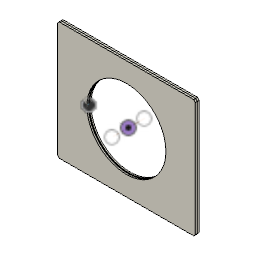
assembly (Autodesk Fusion 360 archive; units mm, degrees)
design "Condensor lens mount"
part number: 2026-06-29-18-31-42-518
Autodesk Fusion 360 part; units mm, degrees
sketch "Sketch1" plane through (0, 0, 0) normal (0, 1, 0) x (1, 0, 0)
  line L0 (87.5, -75) -> (-87.5, -75)
  line L1 (-87.5, -75) -> (-87.5, 75)
  line L2 (-87.5, 75) -> (87.5, 75)
  line L3 (87.5, 75) -> (87.5, -75)
  line L4 (87.5, -75) -> (-87.5, 75) construction
  line L5 (-87.5, -75) -> (87.5, 75) construction
  line L6 (-87.5, -72.7222) -> (-85.5476, -75)
  line L7 (0, -75) -> (0, 75) construction
  line L8 (-87.5, 0) -> (87.5, 0) construction
  line L9 (87.5, -72.7222) -> (85.5476, -75)
  line L10 (87.5, 72.7222) -> (85.5476, 75)
  line L11 (-87.5, 72.7222) -> (-85.5476, 75)
  circle A0 centre (0, 0) radius 50
  dimension "d1" = 175
  dimension "d2" = 150
  dimension "d3" = 3
  dimension "d4" = 100
  constraint horizontal L0
  constraint perpendicular L0 L1
  constraint parallel L0 L2
  constraint parallel L1 L3
  constraint coincident L4 A0.centre
  constraint coincident L5 A0.centre
  constraint coincident A0.centre origin
  constraint coincident L1 L6.start
  constraint coincident L0 L6.end
  constraint perpendicular L5 L6
  constraint midpoint L0 L7.start
  constraint midpoint L2 L7.end
  constraint midpoint L1 L8.start
  constraint midpoint L3 L8.end
  constraint symmetric L6.start L7 L9.start
  constraint symmetric L6.end L7 L9.end
  constraint symmetric L6.start L8 L11.start
  constraint symmetric L6.end L8 L11.end
  constraint symmetric L8 L9.start L10.start
  constraint symmetric L8 L9.end L10.end
  measures "d1" distance of L1.end L2.end
  measures "d2" distance of L0.end L1.end
  measures "d3" distance of L6.start L6.end
  measures "d4" diameter of A0
sketch "Sketch2" plane through (0, 2.5, 0) normal (0, 1, 0) x (1, 0, 0)
sketch "Sketch3" plane through (50, 2.5597, 0) normal (-1, 0, 0) x (0, -1, 0)
sketch "Sketch5" plane through (0, 0, 0) normal (0, 0, 1) x (1, 0, 0)
  line L0 (-50, 0.5) -> (-50, -0.5)
  arc A0 (-50, 0.5) -> (-50, -0.5) centre (-50, 0) ccw
  line L1 (0, 20) -> (0, -21)
  line L2 (-50.5, 0) -> (0, 0) construction
  dimension "d9" = 1
  dimension "d14" = 1
  constraint vertical L0
  constraint midpoint L0 A0.centre
  constraint vertical L1
  constraint midpoint A0 L2.start
  constraint coincident L2.end origin
  constraint perpendicular L1 L2
  measures "d9" distance of L0.start L0.end
  measures "d14" diameter of A0
extrude "Extrude4" add sketch "Sketch1" along normal mid plane 5 contours L0 L1 L2 L3 L6 L9 L10 L11 makes body 1
revolve "Revolve2" cut sketch "Sketch5" angle 360 about axis through (0, 20, 0) along (0, -1, 0) bodies 1
fillet "Fillet1" radius 0.1 2 edges at (-46.6164, 0.5, -18.0808) (-46.6164, -0.5, 18.0808) on bodies 1
split "Split1" by plane through (0, 0, 0) normal (0, 1, 0) bodies 1 makes body 2 at (75, 2.5, 0)

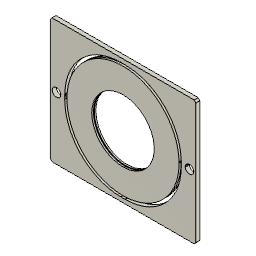
design "Projector Lens mount"
part number: 2026-06-30-17-54-35-923
part number: 2026-08-02-16-02-17-877
part number: 2026-08-02-16-06-35-428
Autodesk Fusion 360 part; units mm, degrees
sketch "Sketch1" plane through (0, 0, 0) normal (0, 1, 0) x (1, 0, 0)
  line L0 (87.5, -75) -> (-87.5, -75)
  line L1 (-87.5, -75) -> (-87.5, 75)
  line L2 (-87.5, 75) -> (87.5, 75)
  line L3 (87.5, 75) -> (87.5, -75)
  line L4 (87.5, -75) -> (-87.5, 75) construction
  line L5 (-87.5, -75) -> (87.5, 75) construction
  circle A0 centre (0, 0) radius 37.5
  line L6 (-87.5, -72.7222) -> (-85.5476, -75)
  line L7 (0, -75) -> (0, 75) construction
  line L8 (-87.5, 0) -> (87.5, 0) construction
  line L9 (87.5, -72.7222) -> (85.5476, -75)
  line L10 (-87.5, 72.7222) -> (-85.5476, 75)
  line L11 (87.5, 72.7222) -> (85.5476, 75)
  circle A1 centre (0, 0) radius 67.5
  line L12 (-69.3129, -70) -> (-70.6939, 70)
  line L13 (-81.6667, -70) -> (-82.5, -70)
  line L14 (-82.5, 70) -> (-81.6667, 70)
  line L15 (69.3129, -70) -> (70.6939, 70)
  line L16 (82.5, -70) -> (81.6667, -70)
  line L17 (69.3129, -70) -> (-69.3129, -70)
  line L18 (-70.6939, 70) -> (70.6939, 70)
  line L19 (81.6667, 70) -> (82.5, 70)
  dimension "d1" = 175
  dimension "d2" = 150
  dimension "d3" = 75
  dimension "d4" = 3
  dimension "d14" = 135
  dimension "d21" = 70
  constraint horizontal L0
  constraint perpendicular L0 L1
  constraint parallel L0 L2
  constraint parallel L1 L3
  constraint coincident L4 A0.centre
  constraint coincident L5 A0.centre
  constraint coincident A0.centre A1.centre
  constraint coincident L1 L6.start
  constraint coincident L0 L6.end
  constraint perpendicular L5 L6
  constraint midpoint L0 L7.start
  constraint midpoint L2 L7.end
  constraint midpoint L1 L8.start
  constraint midpoint L3 L8.end
  constraint symmetric L6.start L7 L9.start
  constraint symmetric L6.end L7 L9.end
  constraint symmetric L6.start L8 L10.start
  constraint symmetric L6.end L8 L10.end
  constraint symmetric L8 L9.start L11.start
  constraint symmetric L8 L9.end L11.end
  constraint concentric A0 A1
  constraint coincident L5 L13.start
  constraint collinear L13 L17
  constraint coincident L4 L14.end
  constraint collinear L14 L18
  constraint symmetric L7 L12.start L15.start
  constraint symmetric L7 L12.end L15.end
  constraint coincident L4 L16.end
  constraint collinear L16 L17
  constraint coincident L5 L19.start
  constraint collinear L18 L19
  measures "d1" distance of L1.end L2.end
  measures "d2" distance of L0.end L1.end
  measures "d3" diameter of A0
  measures "d4" distance of L6.start L6.end
  measures "d14" diameter of A1
  measures "d21" distance of A0.centre L12
extrude "Extrude1" add sketch "Sketch1" along normal mid plane 5 contours L0 L1 L2 L3 L6 L9 L10 L11 | A1 makes body 1 at (75.8356, 2.5, 24.2407) makes body 2 at (57.2487, 2.5, 3.3535)
sketch "Sketch2" plane through (0, 0, 0) normal (0, 0, 1) x (1, 0, 0)
  line L0 (0, 0) -> (38, 0) construction
  line L1 (37.5, 0) -> (37.5, 0.5)
  line L2 (37.5, 0) -> (37.5, -0.5)
  arc A0 (37.5, -0.5) -> (37.5, 0.5) centre (37.5, 0) ccw
  line L3 (0, 25) -> (0, -28)
  dimension "d7" = 38
  dimension "d9" = 1
  dimension "d10" = 0.5
  constraint coincident L0.start origin
  constraint horizontal L0
  constraint coincident L0 L1.start
  constraint coincident L1.start L2.start
  constraint perpendicular L0 L1
  constraint perpendicular L0 L2
  constraint vertical L3
  measures "d7" distance of L0.start L0.end
  measures "d9" diameter of A0
  measures "d10" distance of L0.end L1.start
revolve "Revolve1" cut sketch "Sketch2" angle 360 about axis through (0, 25, 0) along (0, -1, 0) bodies 1
split "Split1" by plane through (0, 0, 0) normal (0, 1, 0) bodies 1 makes body 3 at (75.8356, 2.5, 24.2407)
fillet "Fillet1" [no effect]
revolve "Revolve2" cut sketch "Sketch2" angle 360 about axis through (0, 25, 0) along (0, -1, 0) bodies 2
split "Split2" by plane through (0, 0, 0) normal (0, 1, 0) bodies 2 makes body 4 at (57.2487, 2.5, 3.3535)
sketch "Sketch3" plane through (69.9966, 0, 0.6905) normal (0.999951, 0, 0.009864) x (0, 1, 0)
  line L0 (0, -72.7222) -> (0, 72.7222)
  line L1 (0, 72.7222) -> (-2.5, 72.7222)
  line L2 (-2.5, 72.7222) -> (-2.5, -72.7222)
  line L3 (-2.5, -72.7222) -> (0, -72.7222)
  circle A0 centre (0, 0) radius 1.6
  line L4 (0, 69.3129) -> (0, -70.6939)
  line L5 (0, -70.6939) -> (-2.5, -70.6939)
  line L6 (-2.5, -70.6939) -> (-2.5, 69.3129)
  line L7 (-2.5, 69.3129) -> (0, 69.3129)
  dimension "d23" = 3.2
  constraint coincident A0.centre origin
  measures "d23" diameter of A0
extrude "Extrude2" cut sketch "Sketch3" against normal blind 10 contours L0 A0 L4 | L0 A0 L4 bodies 2 4
extrude "Extrude3" cut sketch "Sketch3" along normal blind 5 contours L0 A0 L4 | L0 A0 L4 bodies 1 3
mirror "Mirror1" about plane through (0, 0, 0) normal (1, 0, 0) of "Extrude2", "Extrude3"
combine "Combine1" operation add target body 1 tool bodies 3
fillet "Fillet2" radius 67.5 1 edges at (-69.3129, 0, 70) on bodies 1
fillet "Fillet3" radius 67.5 3 edges at (69.3129, 0, 70) (70.6939, 0, -70) (-70.6939, 0, -70) on bodies 1
copy_body "CutPasteBodies1" bodies 2 4 removing the originals makes body 5 makes body 6 in component "gYRO"
copy_body "CutPasteBodies1'" bodies 1 removing the originals makes body 7 in component "Frame"
sketch "Sketch4" plane through (0, -2.5, 0) normal (0, -1, 0) x (-0.999792, 0, 0.020411)
  circle A0 centre (0.011, 0.0001) radius 37.5
  circle A1 centre (0.011, 0.0001) radius 67.5
  line L0 (8, 56) -> (-8, 56)
  line L1 (-8, 56) -> (-8, 48)
  line L2 (-8, 48) -> (8, 48)
  line L3 (8, 48) -> (8, 56)
  line L4 (8, 56) -> (-8, 48) construction
  line L5 (-8, 56) -> (8, 48) construction
  point P0 (0, 52)
  dimension "d38" = 8
  constraint horizontal L0
  constraint perpendicular L0 L1
  constraint parallel L0 L2
  constraint parallel L1 L3
  constraint coincident L4 P0
  constraint coincident L5 P0
  measures "d38" distance of L0.end L1.end
sketch "Sketch1 (2)" plane through (0, 2.5, 0) normal (0, 1, 0) x (-1, 0, 0) in component "gYRO"
  circle A0 centre (0, 0) radius 37.5
  circle A1 centre (0, 0) radius 67.5
  line L0 (8, -45) -> (-8, -45)
  line L1 (-8, -45) -> (-8, -53)
  line L2 (-8, -53) -> (8, -53)
  line L3 (8, -53) -> (8, -45)
  line L4 (8, -45) -> (-8, -53) construction
  line L5 (-8, -45) -> (8, -53) construction
  point P0 (0, -49)
  dimension "d39" = 16
  dimension "d40" = 8
  dimension "d41" = 45
  constraint horizontal L0
  constraint perpendicular L0 L1
  constraint parallel L0 L2
  constraint parallel L1 L3
  constraint coincident L4 P0
  constraint coincident L5 P0
  measures "d39" distance of L1.end L2.end
  measures "d40" distance of L0.end L1.end
  measures "d41" distance of A0.centre L0
extrude "Extrude1'" add sketch "Sketch1 (2)" along normal blind 1 contours L0 L1 L2 L3 bodies 6 in component "gYRO"
ref_plane "WorkPlane1" through (8, 3.5, -49) normal (1, 0, 0) x (0, 0, -1) in component "gYRO"
sketch "Sketch2 (2)" plane through (8, 0, 0) normal (1, 0, 0) x (0, 1, 0) in component "gYRO"
  line L0 (3.5, -45) -> (3.5, -53)
  line L1 (3.5, -45) -> (6.75, -45)
  line L2 (9.5, -47.75) -> (9.5, -50.25)
  line L3 (6.75, -53) -> (3.5, -53)
  line L4 (3.5, -53) -> (3.5, -45)
  circle A0 centre (6.5, -49) radius 1.6
  arc A1 (9.5, -47.75) -> (6.75, -45) centre (6.75, -47.75) ccw
  arc A2 (6.75, -53) -> (9.5, -50.25) centre (6.75, -50.25) ccw
  point P0 (9.5, -45)
  dimension "d46" = 6
  dimension "d47" = 3.2
  dimension "d48" = 2.75
  constraint horizontal L1
  constraint vertical L2
  constraint horizontal L3
  constraint vertical L4
  constraint coincident L0.start L1.start
  constraint coincident P0 L1
  constraint coincident P0 L2
  constraint tangent L1 A1
  constraint tangent L2 A1
  constraint tangent L2 A2
  constraint tangent L3 A2
  constraint equal A1 A2
  measures "d46" distance of L0.start P0
  measures "d47" diameter of A0
  measures "d48" radius of A1
extrude "Extrude2'" add sketch "Sketch2 (2)" against normal blind 1 separate body makes body 8 in component "gYRO"
mirror "Mirror1'" about plane through (0.011, 0, -0.0001) normal (1, 0, 0) of bodies 8 makes body 9 in component "gYRO"
combine "Combine1'" operation add target body 6 tool bodies 8 9 in component "gYRO"
sketch "Sketch5" plane through (0, 2.5, 0) normal (0, 1, 0) x (-1, 0, 0)
  line L0 (-70.0215, -1.8342) -> (-69.9722, 3.1658)
  arc A0 (-2.4755, 70) -> (-69.9722, 3.1658) centre (-2.4755, 2.5) ccw
  line L1 (-2.4755, 70) -> (2.4755, 70)
  arc A1 (69.9722, 3.1658) -> (2.4755, 70) centre (2.4755, 2.5) ccw
  line L2 (69.9722, 3.1658) -> (70.0215, -1.8342)
  arc A2 (2.5248, -70) -> (70.0215, -1.8342) centre (2.5248, -2.5) ccw
  line L3 (2.5248, -70) -> (-2.5248, -70)
  arc A3 (-70.0215, -1.8342) -> (-2.5248, -70) centre (-2.5248, -2.5) ccw
  line L4 (-87.5, 72.7222) -> (-87.5, -72.7222)
  line L5 (-87.5, -72.7222) -> (-85.5476, -75)
  line L6 (-85.5476, -75) -> (85.5476, -75)
  line L7 (85.5476, -75) -> (87.5, -72.7222)
  line L8 (87.5, -72.7222) -> (87.5, 72.7222)
  line L9 (87.5, 72.7222) -> (85.5476, 75)
  line L10 (85.5476, 75) -> (-85.5476, 75)
  line L11 (-85.5476, 75) -> (-87.5, 72.7222)
  circle A4 centre (-80, 0) radius 5.1
  line L12 (0, 30) -> (0, -21.7495)
  circle A5 centre (80, 0) radius 5.1
  dimension "d53" = 10.2
  dimension "d54" = 7.5
  dimension "d55" = 75
  constraint vertical L12
  constraint symmetric A4 L12 A5
  measures "d53" diameter of A4
  measures "d54" distance of L4 A4.centre
  measures "d55" distance of L10 A4.centre
extrude "Extrude1''" cut sketch "Sketch5" against normal blind 10 contours A4 | A5 bodies 7 in component "Frame"
component "gYRO" placed x (1, 0, 0) y (0, 1, 0) z (0, 0, 1) at (-0.011, 0, 0.0001)
component "Frame" placed x (1, 0, 0) y (0, 1, 0) z (0, 0, 1) at (0, 0, 0)

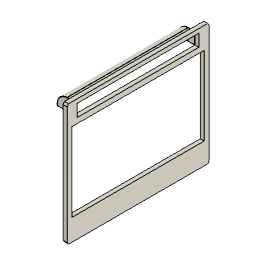
design "LCD mount"
part number: 2026-06-29-18-25-40-189
Autodesk Fusion 360 part; units mm, degrees
sketch "Sketch1" plane through (0, 0, 0) normal (1, 0, 0) x (0, 1, 0)
  line L0 (87.5, 75) -> (-87.5, 75)
  line L1 (-87.5, 75) -> (-87.5, -75)
  line L2 (-87.5, -75) -> (87.5, -75)
  line L3 (87.5, -75) -> (87.5, 75)
  line L4 (87.5, 75) -> (-87.5, -75) construction
  line L5 (-87.5, 75) -> (87.5, -75) construction
  line L6 (-87.5, 72.5134) -> (-85.8217, 75)
  line L7 (0, 75) -> (0, -75) construction
  line L8 (-87.5, 0) -> (87.5, 0) construction
  line L9 (87.5, 72.5134) -> (85.8217, 75)
  line L10 (87.5, -72.5134) -> (85.8217, -75)
  line L11 (-87.5, -72.5134) -> (-85.8217, -75)
  line L12 (81.5, 48.35) -> (-81.5, 48.35)
  line L13 (-81.5, 48.35) -> (-81.5, -48.35)
  line L14 (-81.5, -48.35) -> (81.5, -48.35)
  line L15 (81.5, -48.35) -> (81.5, 48.35)
  line L16 (81.5, 48.35) -> (-81.5, -48.35) construction
  line L17 (-81.5, 48.35) -> (81.5, -48.35) construction
  line L18 (75, 55) -> (-75, 55)
  line L19 (-75, 55) -> (-75, 70)
  line L20 (-75, 70) -> (75, 70)
  line L21 (75, 70) -> (75, 55)
  line L22 (75, 55) -> (-75, 70) construction
  line L23 (-75, 55) -> (75, 70) construction
  point P0 (0, 62.5)
  dimension "d1" = 175
  dimension "d2" = 150
  dimension "d3" = 3
  dimension "d4" = 163
  dimension "d5" = 96.7
  dimension "d8" = 150
  dimension "d9" = 15
  dimension "d10" = 5
  constraint horizontal L0
  constraint perpendicular L0 L1
  constraint parallel L0 L2
  constraint parallel L1 L3
  constraint coincident L4 origin
  constraint coincident L5 origin
  constraint coincident L1 L6.start
  constraint coincident L0 L6.end
  constraint midpoint L0 L7.start
  constraint midpoint L2 L7.end
  constraint midpoint L1 L8.start
  constraint midpoint L3 L8.end
  constraint symmetric L6.start L7 L9.start
  constraint symmetric L6.end L7 L9.end
  constraint symmetric L6.start L8 L11.start
  constraint symmetric L6.end L8 L11.end
  constraint symmetric L8 L9.start L10.start
  constraint symmetric L8 L9.end L10.end
  constraint horizontal L12
  constraint perpendicular L12 L13
  constraint parallel L12 L14
  constraint parallel L13 L15
  constraint coincident L16 origin
  constraint coincident L17 origin
  constraint horizontal L18
  constraint perpendicular L18 L19
  constraint parallel L18 L20
  constraint parallel L19 L21
  constraint coincident L22 P0
  constraint coincident L23 P0
  constraint coincident L7 P0
  measures "d1" distance of L1.end L2.end
  measures "d2" distance of L0.end L1.end
  measures "d3" distance of L6.start L6.end
  measures "d4" distance of L13.end L14.end
  measures "d5" distance of L12.end L13.end
  measures "d8" distance of L19.end L20.end
  measures "d9" distance of L18.end L19.end
  measures "d10" distance of L0 L20
extrude "Extrude1" add sketch "Sketch1" along normal blind 5 contours L0 L1 L2 L3 L6 L9 L10 L11 | L18 L19 L20 L21 makes body 1
extrude "Extrude2" cut sketch "Sketch1" along normal blind 10 contours L18 L19 L20 L21 bodies 1
sketch "Sketch2" plane through (0, 0, 0) normal (-1, 0, 0) x (0, -1, 0)
  line L0 (-75, 55) -> (-75, 70)
  line L1 (-75, 70) -> (75, 70)
  line L2 (75, 70) -> (75, 55)
  line L3 (75, 55) -> (-75, 55)
  line L4 (-81.5, -48.35) -> (-81.5, 48.35)
  line L5 (-81.5, 48.35) -> (81.5, 48.35)
  line L6 (81.5, 48.35) -> (81.5, -48.35)
  line L7 (81.5, -48.35) -> (-81.5, -48.35)
  line L8 (87.5, -72.5134) -> (87.5, 72.5134)
  line L9 (87.5, 72.5134) -> (85.8217, 75)
  line L10 (85.8217, 75) -> (-85.8217, 75)
  line L11 (-85.8217, 75) -> (-87.5, 72.5134)
  line L12 (-87.5, 72.5134) -> (-87.5, -72.5134)
  line L13 (-87.5, -72.5134) -> (-85.8217, -75)
  line L14 (-85.8217, -75) -> (85.8217, -75)
  line L15 (85.8217, -75) -> (87.5, -72.5134)
ref_plane "WorkPlane1" through (0, 75, 0) normal (0, 1, 0) x (0, 0, 1)
sketch "Sketch3" plane through (0, 75, 0) normal (0, 1, 0) x (1, 0, 0)
  line L0 (0, -55) -> (-20, -55)
  line L1 (0, -70) -> (-7.75, -70)
  spline S0 degree 1 poles (-20, -55) (-20, -57.75) knots 0 0 0.183333 0.183333
  arc A0 (-20, -57.75) -> (-7.75, -70) centre (-7.75, -57.75) ccw
  line L2 (-20, -55) -> (-20, -57.75) construction
  line L3 (0, -70) -> (0, -55)
  line L4 (0, -69.5) -> (-7.75, -69.5)
  arc A1 (-19.5, -57.75) -> (-7.75, -69.5) centre (-7.75, -57.75) ccw
  spline S1 degree 1 poles (-19.5, -55) (-19.5, -57.75) knots 0 0 0.275 0.275
  point P0 (0, -70)
  point P1 (0, -55)
  dimension "d14" = 20
  dimension "d15" = 12.25
  dimension "d16" = -0.5
  dimension "d17" = -0.5
  constraint horizontal L0
  constraint coincident P0 L1.start
  constraint horizontal L1
  constraint tangent S0 A0
  constraint tangent L1 A0
  constraint perpendicular L0 L3
  measures "d14" distance of L0.start L0.end
  measures "d15" radius of A0
extrude "Extrude3" add sketch "Sketch3" against normal blind 150 separate body contours L0 L1 S0 A0 L3 L4 A1 S1 makes body 2
extrude "Extrude4" add sketch "Sketch3" against normal blind 0.5 separate body contours L0 L3 L4 A1 S1 makes body 3
mirror "Mirror1" about plane through (0, 0, 0) normal (0, 1, 0) of bodies 3 makes body 4
fillet "Fillet1" radius 0.5 3 edges at (-3.875, 75, 70) (-16.4121, 75, 66.4121) (-20, 75, 56.375) on bodies 2
fillet "Fillet2" radius 0.1 1 edges at (-9.75, 75, 55) on bodies 3
fillet "Fillet3" radius 0.1 2 edges at (-19.8536, 74.8536, 55) (-20, -0.25, 55) on bodies 2
fillet "Fillet4" radius 0.1 1 edges at (-9.75, -75, 55) on bodies 4
fillet "Fillet5" radius 0.1 5 edges at (-3.875, -75, 70) (-16.4121, -75, 66.4121) (-20, -75, 56.425) (-19.9707, -75, 55.0293) (-19.7, -75, 55) on bodies 2
